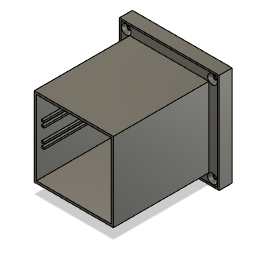
alpha OPC v12 (Autodesk Fusion 360 design; units mm, degrees)
Autodesk Fusion 360 part; units mm, degrees
sketch "Esquisse1" plane through (0, 0, 0) normal (0, 0, 1) x (1, 0, 0)
  line L0 (56.8395, 13.2598) -> (10.8395, 13.2598)
  line L1 (10.8395, 13.2598) -> (10.8395, 59.2598)
  line L2 (10.8395, 59.2598) -> (56.8395, 59.2598)
  line L3 (56.8395, 59.2598) -> (56.8395, 13.2598)
  line L4 (56.8395, 13.2598) -> (10.8395, 59.2598) construction
  line L5 (10.8395, 13.2598) -> (56.8395, 59.2598) construction
  line L6 (62.8395, 7.2598) -> (4.8395, 7.2598)
  line L7 (4.8395, 7.2598) -> (4.8395, 65.2598)
  line L8 (4.8395, 65.2598) -> (62.8395, 65.2598)
  line L9 (62.8395, 65.2598) -> (62.8395, 7.2598)
  line L10 (62.8395, 7.2598) -> (4.8395, 65.2598) construction
  line L11 (4.8395, 7.2598) -> (62.8395, 65.2598) construction
  line L12 (39.3395, 17.2598) -> (27.3395, 17.2598)
  line L13 (27.3395, 17.2598) -> (27.3395, 29.2598)
  line L14 (27.3395, 29.2598) -> (39.3395, 29.2598)
  line L15 (39.3395, 29.2598) -> (39.3395, 17.2598)
  line L16 (39.3395, 17.2598) -> (27.3395, 29.2598) construction
  line L17 (27.3395, 17.2598) -> (39.3395, 29.2598) construction
  circle A0 centre (33.3395, 23.2598) radius 3.05
  circle A1 centre (16.3395, 20.7598) radius 1.15
  circle A2 centre (51.3395, 20.7598) radius 1.15
  line L18 (45.8395, 34.2598) -> (20.8395, 34.2598)
  line L19 (20.8395, 34.2598) -> (20.8395, 49.2598)
  line L20 (20.8395, 49.2598) -> (45.8395, 49.2598)
  line L21 (45.8395, 49.2598) -> (45.8395, 34.2598)
  line L22 (45.8395, 34.2598) -> (20.8395, 49.2598) construction
  line L23 (20.8395, 34.2598) -> (45.8395, 49.2598) construction
  line L24 (55.3395, 14.7598) -> (12.3395, 14.7598)
  line L25 (12.3395, 14.7598) -> (12.3395, 57.7598)
  line L26 (12.3395, 57.7598) -> (55.3395, 57.7598)
  line L27 (55.3395, 57.7598) -> (55.3395, 14.7598)
  line L28 (55.3395, 14.7598) -> (12.3395, 57.7598) construction
  line L29 (12.3395, 14.7598) -> (55.3395, 57.7598) construction
  circle A3 centre (8.7895, 61.3098) radius 1.15
  circle A4 centre (16.3395, 20.7598) radius 3
  line L30 (61.8395, 8.2598) -> (5.8395, 8.2598)
  line L31 (5.8395, 8.2598) -> (5.8395, 64.2598)
  line L32 (5.8395, 64.2598) -> (61.8395, 64.2598)
  line L33 (61.8395, 64.2598) -> (61.8395, 8.2598)
  line L34 (61.8395, 8.2598) -> (5.8395, 64.2598) construction
  line L35 (5.8395, 8.2598) -> (61.8395, 64.2598) construction
  circle A5 centre (51.3395, 20.7598) radius 3
  circle A6 centre (8.7895, 11.2098) radius 1.15
  circle A7 centre (58.8895, 11.2098) radius 1.15
  circle A8 centre (58.8895, 61.3098) radius 1.15
  line L36 (55.5895, 14.5098) -> (12.0895, 14.5098)
  line L37 (12.0895, 14.5098) -> (12.0895, 58.0098)
  line L38 (12.0895, 58.0098) -> (55.5895, 58.0098)
  line L39 (55.5895, 58.0098) -> (55.5895, 14.5098)
  line L40 (55.5895, 14.5098) -> (12.0895, 58.0098) construction
  line L41 (12.0895, 14.5098) -> (55.5895, 58.0098) construction
  line L42 (55.5895, 40.9098) -> (54.0895, 40.9098)
  line L43 (54.0895, 40.9098) -> (54.0895, 39.9098)
  line L44 (54.0895, 39.9098) -> (55.5895, 39.9098)
  line L45 (55.5895, 39.9098) -> (55.5895, 40.9098)
  line L46 (55.5895, 42.6098) -> (54.0895, 42.6098)
  line L47 (54.0895, 42.6098) -> (54.0895, 43.6098)
  line L48 (54.0895, 43.6098) -> (55.5895, 43.6098)
  line L49 (55.5895, 43.6098) -> (55.5895, 42.6098)
  line L50 (55.5895, 32.1824) -> (54.0895, 32.1824)
  line L51 (54.0895, 30.4824) -> (54.0895, 29.4824)
  line L52 (55.5895, 30.4824) -> (54.0895, 30.4824)
  line L53 (54.0895, 32.1824) -> (54.0895, 33.1824)
  line L54 (55.5895, 29.4824) -> (55.5895, 30.4824)
  line L55 (54.0895, 29.4824) -> (55.5895, 29.4824)
  line L56 (54.0895, 33.1824) -> (55.5895, 33.1824)
  line L57 (55.5895, 33.1824) -> (55.5895, 32.1824)
  line L58 (13.5895, 30.5078) -> (12.0895, 30.5078)
  line L59 (12.0895, 30.5078) -> (12.0895, 29.5078)
  line L60 (13.5895, 33.2078) -> (13.5895, 32.2078)
  line L61 (12.0895, 29.5078) -> (13.5895, 29.5078)
  line L62 (13.5895, 32.2078) -> (12.0895, 32.2078)
  line L63 (13.5895, 29.5078) -> (13.5895, 30.5078)
  line L64 (12.0895, 32.2078) -> (12.0895, 33.2078)
  line L65 (12.0895, 33.2078) -> (13.5895, 33.2078)
  line L66 (12.0895, 40.2881) -> (13.5895, 40.2881)
  line L67 (12.0895, 41.2881) -> (12.0895, 40.2881)
  line L68 (12.0895, 43.9881) -> (13.5895, 43.9881)
  line L69 (13.5895, 43.9881) -> (13.5895, 42.9881)
  line L70 (13.5895, 42.9881) -> (12.0895, 42.9881)
  line L71 (13.5895, 40.2881) -> (13.5895, 41.2881)
  line L72 (12.0895, 42.9881) -> (12.0895, 43.9881)
  line L73 (13.5895, 41.2881) -> (12.0895, 41.2881)
  line L74 (54.0895, 32.1824) -> (54.0895, 30.4824)
  line L75 (54.0895, 42.6098) -> (54.0895, 40.9098)
  line L76 (13.5895, 42.9881) -> (13.5895, 41.2881)
  line L77 (13.5895, 32.2078) -> (13.5895, 30.5078)
  line L78 (48.8395, 31.2598) -> (17.8395, 31.2598)
  line L79 (17.8395, 31.2598) -> (17.8395, 52.2598)
  line L80 (17.8395, 52.2598) -> (48.8395, 52.2598)
  line L81 (48.8395, 52.2598) -> (48.8395, 31.2598)
  line L82 (48.8395, 31.2598) -> (17.8395, 52.2598) construction
  line L83 (17.8395, 31.2598) -> (48.8395, 52.2598) construction
  point P0 (33.8395, 36.2598)
  point P1 (33.8395, 36.2598)
  point P2 (33.3395, 23.2598)
  point P3 (33.3395, 41.7598)
  point P4 (33.8395, 36.2598)
  point P5 (33.8395, 36.2598)
  point P6 (33.3395, 41.7598)
  point P7 (33.8395, 36.2598)
  point P8 (33.3395, 41.7598)
  dimension "d2" = 46
  dimension "d10" = 12
  dimension "d11" = 12
  dimension "d12" = 6.1
  dimension "d20" = 2.3
  dimension "d21" = 2.3
  dimension "d23" = 25
  dimension "d24" = 15
  dimension "d36" = 2.3
  dimension "d39" = 6
  dimension "d70" = 2.95
  dimension "d71" = 2.95
  dimension "d80" = 6
  dimension "d84" = 5
  dimension "d86" = 1
  dimension "d87" = 4
  dimension "d92" = 4
  dimension "d95" = 2.3
  dimension "d96" = 2.95
  dimension "d97" = 2.95
  dimension "d98" = 2.3
  dimension "d99" = 2.95
  dimension "d100" = 2.95
  dimension "d101" = 2.3
  dimension "d102" = 2.95
  dimension "d103" = 2.95
  dimension "d109" = 5
  dimension "d110" = 1
  dimension "d111" = 46
  dimension "d112" = 21
  dimension "d114" = 1.25
  dimension "d115" = 0.25
  dimension "d116" = 0.25
  dimension "d117" = 1.25
  dimension "d141" = 1.5
  dimension "d142" = 1
  dimension "d143" = 1.5
  dimension "d144" = 1
  dimension "d145" = 1.7
  dimension "d150" = 21
  dimension "d151" = 6
  dimension "d152" = 16
  dimension "d153" = 6
  dimension "d154" = 15.15
  dimension "d155" = 1.5
  dimension "d156" = 1
  dimension "d157" = 1.5
  dimension "d158" = 1
  dimension "d159" = 1.7
  dimension "d160" = 1.5
  dimension "d161" = 1
  dimension "d162" = 1.5
  dimension "d163" = 1
  dimension "d164" = 1.7
  dimension "d165" = 1.5
  dimension "d166" = 1
  dimension "d167" = 1.5
  dimension "d168" = 1
  dimension "d169" = 1.7
  dimension "d177" = 3
  dimension "d178" = 3
  dimension "d179" = 8.5
  constraint horizontal L0
  constraint perpendicular L0 L1
  constraint parallel L0 L2
  constraint parallel L1 L3
  constraint coincident L4 P7
  constraint coincident L5 P7
  constraint horizontal L6
  constraint perpendicular L6 L7
  constraint parallel L6 L8
  constraint parallel L7 L9
  constraint coincident L10 P7
  constraint coincident L11 P7
  constraint coincident P7 P4
  constraint horizontal L12
  constraint perpendicular L12 L13
  constraint parallel L12 L14
  constraint parallel L13 L15
  constraint coincident L16 P2
  constraint coincident L17 P2
  constraint coincident P2 A0.centre
  constraint horizontal L18
  constraint perpendicular L18 L19
  constraint parallel L18 L20
  constraint parallel L19 L21
  constraint coincident L22 P8
  constraint coincident L23 P8
  constraint horizontal L24
  constraint perpendicular L24 L25
  constraint parallel L24 L26
  constraint parallel L25 L27
  constraint coincident L28 P7
  constraint coincident L29 P7
  constraint coincident P7 P5
  constraint concentric A1 A4
  constraint horizontal L30
  constraint perpendicular L30 L31
  constraint parallel L30 L32
  constraint parallel L31 L33
  constraint coincident L34 P7
  constraint coincident L35 P7
  constraint coincident P8 P6
  constraint concentric A2 A5
  constraint horizontal L36
  constraint perpendicular L36 L37
  constraint parallel L36 L38
  constraint parallel L37 L39
  constraint coincident L4 L36.start
  constraint coincident L40 P7
  constraint coincident L41 P7
  constraint horizontal L42
  constraint vertical L43
  constraint horizontal L44
  constraint vertical L45
  constraint coincident L39 L42.start
  constraint horizontal L46
  constraint vertical L47
  constraint horizontal L48
  constraint vertical L49
  constraint coincident L39 L46.start
  constraint horizontal L52
  constraint vertical L51
  constraint horizontal L55
  constraint vertical L54
  constraint horizontal L50
  constraint vertical L53
  constraint horizontal L56
  constraint vertical L57
  constraint horizontal L58
  constraint vertical L59
  constraint horizontal L61
  constraint vertical L63
  constraint horizontal L62
  constraint vertical L64
  constraint horizontal L65
  constraint vertical L60
  constraint horizontal L73
  constraint vertical L67
  constraint horizontal L66
  constraint vertical L71
  constraint horizontal L70
  constraint vertical L72
  constraint horizontal L68
  constraint vertical L69
  constraint perpendicular L52 L74
  constraint perpendicular L73 L76
  constraint perpendicular L58 L77
  constraint horizontal L78
  constraint perpendicular L78 L79
  constraint parallel L78 L80
  constraint parallel L79 L81
  constraint coincident L82 P8
  constraint coincident L83 P8
  constraint coincident L37 L64.end
  constraint coincident L37 L68.start
  constraint coincident L39 L56.end
  measures "d2" distance of L0.end L1.end
  measures "d10" distance of L13.end L14.end
  measures "d11" distance of L12.end L13.end
  measures "d12" diameter of A0
  measures "d20" diameter of A1
  measures "d21" diameter of A2
  measures "d23" distance of L19.end L20.end
  measures "d24" distance of L18.end L19.end
  measures "d36" diameter of A3
  measures "d39" diameter of A4
  measures "d70" distance of A3.centre L32
  measures "d71" distance of A3.centre L31
  measures "d80" diameter of A5
  measures "d84" distance of L2 L32
  measures "d86" distance of L8 L32
  measures "d87" distance of L25 A1.centre
  measures "d92" distance of L27 A2.centre
  measures "d95" diameter of A6
  measures "d96" distance of L30 A6.centre
  measures "d97" distance of L31 A6.centre
  measures "d98" diameter of A7
  measures "d99" distance of L30 A7.centre
  measures "d100" distance of L33 A7.centre
  measures "d101" diameter of A8
  measures "d102" distance of L32 A8.centre
  measures "d103" distance of L33 A8.centre
  measures "d109" distance of L1 L31
  measures "d110" distance of L7 L31
  measures "d111" distance of L1.end L2.end
  measures "d112" distance of P2 L25
  measures "d114" distance of L1 L37
  measures "d115" distance of L25 L37
  measures "d116" distance of L26 L38
  measures "d117" distance of L2 L38
  measures "d141" distance of L42.start L42.end
  measures "d142" distance of L42.start L44.end
  measures "d143" distance of L46.start L46.end
  measures "d144" distance of L46.start L48.end
  measures "d145" distance of L42 L46
  measures "d150" distance of P8 L25
  measures "d151" distance of A1.centre L24
  measures "d152" distance of L26 P8
  measures "d153" distance of A2.centre L24
  measures "d154" distance of L26 L46.end
  measures "d155" distance of L51.start L52.start
  measures "d156" distance of L52.start L54.start
  measures "d157" distance of L50.start L50.end
  measures "d158" distance of L56.end L50.start
  measures "d159" distance of L50 L52
  measures "d160" distance of L58.start L58.end
  measures "d161" distance of L58.start L61.end
  measures "d162" distance of L62.end L60.end
  measures "d163" distance of L60.end L60.start
  measures "d164" distance of L58 L62
  measures "d165" distance of L67.start L71.end
  measures "d166" distance of L71.end L66.end
  measures "d167" distance of L69.end L70.end
  measures "d168" distance of L68.end L69.end
  measures "d169" distance of L70 L73
  measures "d177" distance of L20 L80
  measures "d178" distance of L19 L79
  measures "d179" distance of P2 L24
extrude "Extrusion8" add sketch "Esquisse1" along normal blind 1 contours L0 L1 L2 L3 | L12 L13 L14 L15 | A1 | A2 | L24 L25 L27 L36 L37 L39 L55 L61 | L24 L25 L26 L27 L43 L44 L47 L48 L51 L53 L55 L56 L60 L61 L63 L65 L66 L68 L69 L71 L74 L75 L76 L77 | L27 L51 L52 L55 | L27 L39 L52 L54 L55 | L25 L37 L58 L59 L61 | L25 L58 L61 L63 | L27 L50 L52 L74 | L27 L39 L50 L52 | L25 L37 L58 L62 | L25 L58 L62 L77 | L27 L50 L53 L56 | L27 L39 L50 L56 L57 | L25 L37 L62 L64 L65 | L25 L60 L62 L65 | L27 L39 L44 L56 | L25 L37 L65 L66 | L27 L42 L43 L44 | L27 L39 L42 L44 L45 | L25 L37 L66 L67 L73 | L25 L66 L71 L73 | L27 L42 L46 L75 | L27 L39 L42 L46 | L25 L37 L70 L73 | L25 L70 L73 L76 | L27 L46 L47 L48 | L27 L39 L46 L48 L49 | L25 L37 L68 L70 L72 | L25 L68 L69 L70 | L25 L26 L27 L37 L38 L39 L48 L68 | A3 | A4 | L30 L31 L32 L33 | A5 | A6 | A7 | A8 | L78 L79 L80 L81 makes body 1
extrude "Extrusion26" add sketch "Esquisse1" along normal blind 7.5 contours L6 L7 L8 L9 bodies 1
extrude "Extrusion27" add sketch "Esquisse1" along normal blind 5.5 contours L30 L31 L32 L33 bodies 1
extrude "Extrusion29" add sketch "Esquisse1" along normal blind 3 contours L0 L1 L2 L3 | L12 L13 L14 L15 | L24 L25 L27 L36 L37 L39 L55 L61 | L24 L25 L26 L27 L43 L44 L47 L48 L51 L53 L55 L56 L60 L61 L63 L65 L66 L68 L69 L71 L74 L75 L76 L77 | L27 L51 L52 L55 | L27 L39 L52 L54 L55 | L25 L37 L58 L59 L61 | L25 L58 L61 L63 | L27 L50 L52 L74 | L27 L39 L50 L52 | L25 L37 L58 L62 | L25 L58 L62 L77 | L27 L50 L53 L56 | L27 L39 L50 L56 L57 | L25 L37 L62 L64 L65 | L25 L60 L62 L65 | L27 L39 L44 L56 | L25 L37 L65 L66 | L27 L42 L43 L44 | L27 L39 L42 L44 L45 | L25 L37 L66 L67 L73 | L25 L66 L71 L73 | L27 L42 L46 L75 | L27 L39 L42 L46 | L25 L37 L70 L73 | L25 L70 L73 L76 | L27 L46 L47 L48 | L27 L39 L46 L48 L49 | L25 L37 L68 L70 L72 | L25 L68 L69 L70 | L25 L26 L27 L37 L38 L39 L48 L68 bodies 1
extrude "Extrusion30" add sketch "Esquisse1" along normal blind 15 contours A4 | A5 bodies 1
extrude "Extrusion21" add sketch "Esquisse1" along normal blind 4 from surface at 3.5 separate body contours L30 L31 L32 L33 makes body 2
extrude "Extrusion22" add sketch "Esquisse1" along normal blind 60 from surface at 3 contours L0 L1 L2 L3 bodies 2
extrude "Extrusion24" add sketch "Esquisse1" along normal blind 40 from surface at 20 contours L27 L51 L52 L55 | L27 L39 L52 L54 L55 | L25 L37 L58 L59 L61 | L25 L58 L61 L63 | L27 L50 L53 L56 | L27 L39 L50 L56 L57 | L25 L37 L62 L64 L65 | L25 L60 L62 L65 | L27 L42 L43 L44 | L27 L39 L42 L44 L45 | L25 L37 L66 L67 L73 | L25 L66 L71 L73 | L27 L46 L47 L48 | L27 L39 L46 L48 L49 | L25 L37 L68 L70 L72 | L25 L68 L69 L70 bodies 2
extrude "Extrusion25" add sketch "Esquisse1" along normal blind 2 from surface at 20 contours L27 L50 L52 L74 | L27 L39 L50 L52 | L25 L37 L58 L62 | L25 L58 L62 L77 | L27 L42 L46 L75 | L27 L39 L42 L46 | L25 L37 L70 L73 | L25 L70 L73 L76 bodies 2
chamfer "Chanfrein4" distance 1.65 angle 45 4 edges at (7.7173, 61.7257, 7.5) (7.7173, 11.6257, 7.5) (57.8173, 61.7257, 7.5) (57.8173, 11.6257, 7.5) on bodies 2
chamfer "Chanfrein5" distance 1 angle 45 4 edges at (33.3395, 49.2598, 0) (45.8395, 41.7598, 0) (33.3395, 34.2598, 0) (20.8395, 41.7598, 0) on bodies 1
equation "d20 = diam_autotaraudage"
equation "d21 = diam_autotaraudage"
equation "d36 = diam_autotaraudage"
equation "d95 = diam_autotaraudage"
equation "d98 = diam_autotaraudage"
equation "d101 = diam_autotaraudage"
equation "hauteur = 48 mm"
equation "diam_autotaraudage = 2.3 mm"
